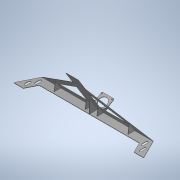
# Autodesk Inventor part: Suporte_Motor
Saved by Autodesk Inventor 2022 (Build 260153000, 153)
## iProperties
Manager: Standard
Created: 2016-02-21
Part Number: Suporte_Motor
Material: SAE 1010/1020
Document SubType Name: Modeling
Designer: Everton
Authority: Rafael Salvador
Manufacturer: Standard
Standards Organization: Custom
Density: 7.86 g/cm^3
Appearance: Steel
Mass: 19558.2 g
Surface Area: 2597.77 cm^2
Volume: 2488.33 cm^3
Author: Everton
Comments: -
Revision Number: 00
Autodesk Inventor part; units mm, degrees
ref_plane "YZ Plane" through (0, 0, 0) normal (1, 0, 0) x (0, 1, 0)
ref_plane "XZ Plane" through (0, 0, 0) normal (0, 1, 0) x (-1, 0, 0)
ref_plane "XY Plane" through (0, 0, 0) normal (0, 0, 1) x (1, 0, 0)
sketch "Sketch1" plane through (0, 0, 0) normal (0, 0, 1) x (1, 0, 0)
  line L0 (9.7407, 1114.2593) -> (159.7407, 1114.2593)
  line L1 (9.7407, 1114.2593) -> (-140.2593, 1114.2593)
  line L2 (-290.2593, 814.2593) -> (-140.2593, 1114.2593)
  line L3 (159.7407, 1114.2593) -> (459.7407, 514.2593)
  line L4 (135.0194, 1074.2593) -> (9.7407, 1074.2593)
  line L5 (9.7407, 1074.2593) -> (-115.5379, 1074.2593)
  line L6 (-115.5379, 1074.2593) -> (-245.5379, 814.2593)
  line L7 (9.7407, 1114.2593) -> (159.7407, 1114.2593)
  line L8 (9.7407, 1114.2593) -> (-140.2593, 1114.2593)
  line L9 (-440.2593, 514.2593) -> (-140.2593, 1114.2593)
  line L10 (159.7407, 1114.2593) -> (309.9483, 813.8441)
  line L11 (135.0194, 1074.2593) -> (9.7407, 1074.2593)
  line L12 (9.7407, 1074.2593) -> (-115.5379, 1074.2593)
  line L13 (-115.5379, 1074.2593) -> (-245.5379, 814.2593)
  line L14 (-245.5379, 814.2593) -> (-290.2593, 814.2593)
  line L15 (265.227, 813.8441) -> (309.9483, 813.8441)
  line L16 (265.227, 813.8441) -> (135.0194, 1074.2593)
  line L17 (415.0194, 514.2593) -> (135.0194, 1074.2593)
  line L18 (-395.5379, 514.2593) -> (-440.2593, 514.2593)
  line L19 (-245.5379, 814.2593) -> (-395.5379, 514.2593)
  line L20 (-440.2593, 514.2593) -> (-395.5379, 514.2593)
  line L21 (415.0194, 514.2593) -> (459.7407, 514.2593)
  point P0 (0, 0)
  dimension "d13" = 300
  constraints: 44 end point, 4 horizontal, 2 point on line, 1 midpoint
  measures "d13" distance from line of L6.end L1
extrude "Extrusion1" add sketch "Sketch1" along normal blind 40 contours L0 L3 L15 L16 L4 L5 L6 L14 L2 L1
extrude "Extrusion3" add sketch "Sketch1" along normal blind 40 contours L3 L21 L17 L15 | L14 L19 L18 L9
sketch "Esboço5" plane through (0, 0, 0) normal (0, 0, 1) x (1, 0, 0)
  line L0 (159.7407, 1114.2593) -> (-140.2593, 1114.2593) projected
  line L1 (400, 897.6863) -> (-384.1407, 897.6863)
  line L2 (-140.2593, 1114.2593) -> (-440.2593, 514.2593) projected
  line L3 (-248.5458, 897.6863) -> (-293.2671, 808.2435)
  line L4 (-395.5379, 514.2593) -> (-115.5379, 1074.2593) projected
  line L5 (-203.8244, 897.6863) -> (-248.5458, 808.2435)
  line L6 (-248.5458, 808.2435) -> (-293.2671, 808.2435)
  line L7 (135.0194, 1074.2593) -> (415.0194, 514.2593) projected
  line L8 (223.3059, 897.6863) -> (268.0272, 808.2435)
  line L9 (459.7407, 514.2593) -> (159.7407, 1114.2593) projected
  line L10 (268.0272, 897.6863) -> (312.7486, 808.2435)
  line L11 (312.7486, 808.2435) -> (268.0272, 808.2435)
  line L12 (-248.5458, 897.6863) -> (312.7486, 897.6863)
  line L13 (312.7486, 897.6863) -> (312.7486, 1190.7632)
  line L14 (312.7486, 1190.7632) -> (-248.5458, 1190.7632)
  line L15 (-248.5458, 1190.7632) -> (-248.5458, 897.6863)
  line L16 (-440.2593, 514.2593) -> (459.7407, 514.2593)
  line L17 (459.7407, 514.2593) -> (459.7407, 808.2435)
  line L18 (459.7407, 808.2435) -> (-440.2593, 808.2435)
  line L19 (-440.2593, 808.2435) -> (-440.2593, 514.2593)
  point P0 (0, 0)
  dimension "d26" = 100
  dimension "d27" = 100
  dimension "d28" = 100
  dimension "d29" = 100
  constraints: 30 end point, 12 point on line, 4 parallel, 3 horizontal, 2 perpendicular
  measures "d26" distance of L3.start L3.end
  measures "d27" distance of L5.start L5.end
  measures "d28" distance of L8.start L8.end
  measures "d29" distance of L10.start L10.end
extrude "Extrusão5" cut sketch "Esboço5" along normal mid plane 100 contours L9 L1 L2 L0 | L0 L2 L15 L14 L13 L1 L9 | L18 L17 L9 | L9 L16 L7 L11 | L6 L4 L16 L2 | L2 L19 L18 | L7 L16 L4 L18
sketch "Esboço6" plane through (0, 0, 0) normal (1, 0, 0) x (0, 1, 0)
  line L0 (897.6863, 40) -> (897.6863, 0) projected
  line L1 (808.2435, 0) -> (808.2435, 40) projected
  line L2 (897.6863, 0) -> (808.2435, 0)
  line L3 (808.2435, 0) -> (808.2435, 1.5)
  line L4 (808.2435, 1.5) -> (897.6863, 1.5)
  line L5 (897.6863, 1.5) -> (897.6863, 0)
  line L6 (808.2435, 1.5) -> (899.6472, 1.5)
  line L7 (899.6472, 1.5) -> (899.6472, 42.2071)
  line L8 (899.6472, 42.2071) -> (808.2435, 42.2071)
  line L9 (808.2435, 42.2071) -> (808.2435, 1.5)
  point P0 (0, 0)
  dimension "d32" = 1.5
  constraints: 16 end point, 4 parallel, 2 horizontal, 2 perpendicular, 1 point on line
  measures "d32" distance of L2.end L3.end
extrude "Extrusão6" cut sketch "Esboço6" along normal mid plane 1000 contours L4 L1 L9 L8 L7 L6
sketch "Esboço28" plane through (0, 0, 0) normal (0, 0, 1) x (1, 0, 0)
  line L0 (223.3059, 897.6863) -> (268.0272, 897.6863) projected
  line L1 (268.0272, 897.6863) -> (253.0272, 897.6863)
  line L2 (28.5, 847.4167) -> (268.0272, 897.6862) projected
  line L3 (268.0272, 897.6862) -> (258.0272, 897.6863)
  line L4 (258.0272, 897.6863) -> (258.0272, 882.6863)
  line L5 (258.0272, 882.6863) -> (258.0272, 877.6863)
  arc A0 (263.0272, 877.6863) -> (253.0272, 877.6863) centre (258.0272, 877.6863) ccw
  line L6 (258.0272, 852.6863) -> (258.0272, 857.6863)
  arc A1 (253.0272, 857.6863) -> (263.0272, 857.6863) centre (258.0272, 857.6863) ccw
  line L7 (263.0272, 877.6863) -> (263.0272, 857.6863)
  line L8 (253.0272, 877.6863) -> (253.0272, 857.6863)
  line L9 (-248.5458, 897.6862) -> (-28.5, 847.8855) projected
  line L10 (-248.5458, 897.6862) -> (-238.5458, 897.6862)
  line L11 (-203.8244, 897.6862) -> (-248.5458, 897.6862) projected
  line L12 (-238.5458, 897.6862) -> (-238.5458, 882.6862)
  line L13 (-238.5458, 882.6862) -> (-238.5458, 877.6862)
  line L14 (-238.5458, 862.6862) -> (-238.5458, 857.6862)
  line L15 (-238.5458, 857.6862) -> (-238.5458, 852.6862)
  arc A2 (-243.5458, 857.6862) -> (-233.5458, 857.6862) centre (-238.5458, 857.6862) ccw
  arc A3 (-233.5458, 877.6862) -> (-243.5458, 877.6862) centre (-238.5458, 877.6862) ccw
  line L16 (-233.5458, 877.6862) -> (-233.5458, 857.6862)
  line L17 (-243.5458, 877.6862) -> (-243.5458, 857.6862)
  line L18 (258.0272, 882.6863) -> (258.0272, 872.6863)
  line L19 (258.0272, 862.6863) -> (258.0272, 852.6863)
  line L20 (268.0272, 808.2435) -> (223.3059, 897.6863) projected
  line L21 (268.0272, 808.2435) -> (278.0272, 808.2435)
  line L22 (312.7486, 808.2435) -> (268.0272, 808.2435) projected
  line L23 (278.0272, 808.2435) -> (278.0272, 813.2435)
  line L24 (278.0272, 813.2435) -> (278.0272, 823.2435)
  line L25 (278.0272, 823.2435) -> (278.0272, 828.2435)
  line L26 (278.0272, 848.2435) -> (278.0272, 853.2435)
  arc A4 (283.0272, 848.2435) -> (273.0272, 848.2435) centre (278.0272, 848.2435) ccw
  arc A5 (273.0272, 828.2435) -> (283.0272, 828.2435) centre (278.0272, 828.2435) ccw
  line L27 (283.0272, 848.2435) -> (283.0272, 828.2435)
  line L28 (273.0272, 848.2435) -> (273.0272, 828.2435)
  line L29 (278.0272, 828.2435) -> (278.0272, 833.2435)
  line L30 (278.0272, 843.2435) -> (278.0272, 848.2435)
  line L31 (-293.2671, 808.2435) -> (-283.2671, 808.2435)
  line L32 (-248.5458, 808.2435) -> (-258.5458, 808.2435)
  line L33 (-248.5458, 808.2435) -> (268.0272, 808.2435) projected
  line L34 (-258.5458, 808.2435) -> (-258.5458, 823.2435)
  line L35 (-258.5458, 823.2435) -> (-258.5458, 828.2435)
  line L36 (-258.5458, 848.2435) -> (-258.5458, 853.2435)
  arc A6 (-253.5458, 848.2435) -> (-263.5458, 848.2435) centre (-258.5458, 848.2435) ccw
  arc A7 (-263.5458, 828.2435) -> (-253.5458, 828.2435) centre (-258.5458, 828.2435) ccw
  line L37 (-253.5458, 848.2435) -> (-253.5458, 828.2435)
  line L38 (-263.5458, 848.2435) -> (-263.5458, 828.2435)
  line L39 (-258.5458, 828.2435) -> (-258.5458, 833.2435)
  line L40 (-258.5458, 843.2435) -> (-258.5458, 848.2435)
  point P0 (0, 0)
  dimension "d126" = 10
  dimension "d127" = 15
  dimension "d128" = 30
  dimension "d129" = 5
  dimension "d130" = 10
  dimension "d131" = 5
  dimension "d132" = 10
  dimension "d133" = 10
  dimension "d134" = 15
  dimension "d135" = 5
  dimension "d136" = 20
  dimension "d137" = 5
  dimension "d138" = 10
  dimension "d139" = 10
  dimension "d140" = 10
  dimension "d143" = 5
  dimension "d144" = 20
  dimension "d145" = 5
  dimension "d146" = 10
  dimension "d147" = 10
  dimension "d149" = 10
  dimension "d151" = 15
  dimension "d152" = 20
  dimension "d153" = 5
  dimension "d154" = 10
  dimension "d155" = 10
  constraints: 68 end point, 20 point on circle, 13 point on line, 8 centre point, 8 coincident, 6 tangent, 4 vertical, 3 perpendicular, 2 midpoint, 1 parallel
  measures "d126" distance of L2.end L3.end
  measures "d127" distance of L3.end L4.end
  measures "d128" distance of L4.end L6.start
  measures "d129" distance of L4.end L5.end
  measures "d130" diameter of A0
  measures "d131" distance of L6.start L6.end
  measures "d132" diameter of A1
  measures "d133" distance of L9.start L10.end
  measures "d134" distance of L10.end L12.end
  measures "d135" distance of L12.end L13.end
  measures "d136" distance of L13.end L14.end
  measures "d137" distance of L14.end L15.end
  measures "d138" diameter of A2
  measures "d139" diameter of A3
  measures "d140" distance of L20.start L21.end
  measures "d143" distance of L24.end L25.end
  measures "d144" distance of L25.end L26.start
  measures "d145" distance of L26.start L26.end
  measures "d146" diameter of A4
  measures "d147" diameter of A5
  measures "d149" distance of L32.start L32.end
  measures "d151" distance of L32.end L34.end
  measures "d152" distance of L35.end L36.start
  measures "d153" distance of L36.start L36.end
  measures "d154" diameter of A6
  measures "d155" diameter of A7
extrude "Extrusão24" cut sketch "Esboço28" along normal mid plane 1000 contours L7 A1 L8 A0 | L17 A3 L16 A2 | L27 A5 L28 A4 | L37 A7 L38 A6
sketch "Esboço35" plane through (0, 0, 0) normal (1, 0, 0) x (0, 1, 0)
  line L0 (0, -158.5228) -> (0, 0) projected
  line L1 (0, 0) -> (0, -158.5228)
  line L2 (0, -158.5228) -> (796.9187, -158.5228) projected
  line L3 (0, -158.5228) -> (796.9187, -158.5228)
  line L4 (895.5819, 0) -> (876.9102, -30) projected
  line L5 (796.9187, -158.5228) -> (895.5819, 0)
  line L6 (895.5819, 0) -> (0, 0)
  line L7 (0, 0) -> (0, -158.5228)
  constraints: 10 end point, 2 perpendicular, 1 collinear, 1 parallel, 1 vertical
extrude "Extrusão29" cut sketch "Esboço35" along normal mid plane 1000
sketch "Esboço42" plane through (0, 0, 0) normal (0, 0, 1) x (1, 0, 0)
  line L0 (223.3059, 897.6863) -> (268.0272, 808.2435) projected
  line L1 (268.0272, 808.2435) -> (223.3059, 897.6863) projected
  line L2 (223.3059, 897.6863) -> (243.1274, 858.0433)
  line L3 (-248.5458, 808.2435) -> (-203.8244, 897.6863) projected
  line L4 (-203.8258, 897.6835) -> (-223.8244, 857.6863)
  line L5 (-203.8244, 897.6863) -> (-248.5458, 808.2435) projected
  line L6 (-203.8244, 897.6863) -> (223.3059, 897.6863)
  line L7 (223.3059, 857.6863) -> (243.3059, 857.6863)
  line L8 (243.3059, 857.6863) -> (-223.8244, 857.6863)
  line L9 (243.3059, 857.6863) -> (223.3059, 897.6863)
  point P0 (0, 0)
  point P1 (224.3581, 895.5819)
  point P2 (-204.8766, 895.5819)
  point P3 (-203.8258, 897.6835)
  dimension "d208" = 40
  constraints: 12 end point, 4 collinear, 3 point on line, 2 horizontal
  measures "d208" distance of L0.start L7.start
extrude "Extrusão33" add sketch "Esboço42" along normal blind 1.5
sketch "Esboço67" plane through (0, 0, 0) normal (0, 1, 0) x (-1, 0, 0)
  line L0 (248.5458, 0) -> (-268.0272, 0) projected
  line L1 (0, 0) -> (248.5458, 0)
  line L2 (-312.7486, 0) -> (-268.0272, 0) projected
  line L3 (248.5458, 0) -> (-268.0272, 0)
  line L4 (0, 0) -> (248.546, 0)
  line L5 (248.546, 0) -> (-9.7405, 0)
  line L6 (-9.7405, 0) -> (-9.7405, 130)
  line L7 (248.5458, 1.5) -> (248.5458, 0) projected
  line L8 (248.5458, 1.5) -> (-268.0272, 1.5) projected
  line L9 (216.6373, 1.5) -> (248.5458, 1.5)
  line L10 (-268.0272, 1.5) -> (-250.4929, 1.5)
  line L11 (-9.7407, 1.5) -> (18.7593, 1.5)
  line L12 (18.7593, 1.5) -> (-38.2407, 1.5)
  line L13 (-38.2407, 1.5) -> (-38.2407, 193.5)
  line L14 (-38.2407, 193.5) -> (18.7593, 193.5)
  line L15 (18.7593, 193.5) -> (18.7593, 1.5)
  line L16 (248.5458, 1.5) -> (203.8418, 1.5)
  line L17 (203.8418, 1.5) -> (-9.7405, 130)
  line L18 (-268.0272, 1.5) -> (-223.3232, 1.5)
  line L19 (-223.3232, 1.5) -> (-9.7405, 130)
  line L20 (248.5458, 1.5) -> (-9.7405, 156.3842)
  line L21 (-268.0272, 1.5) -> (-312.7486, 1.5) projected
  line L22 (-9.7405, 156.3842) -> (-268.0272, 1.5)
  line L23 (146.5111, 1.5) -> (146.5111, 31.5)
  line L24 (146.5111, 31.5) -> (153.9782, 31.5)
  line L25 (-173.4596, 31.5) -> (146.5111, 31.5)
  line L26 (153.9782, 31.5) -> (203.8418, 1.5)
  line L27 (203.8418, 1.5) -> (-223.3232, 1.5)
  line L28 (-223.3232, 1.5) -> (-173.4596, 31.5)
  point P0 (-38.2407, 139.2938)
  point P1 (-38.2407, 112.8531)
  point P2 (18.7593, 139.294)
  point P3 (18.7593, 112.8534)
  point P4 (18.7593, 31.5)
  point P5 (-38.2407, 31.5)
  dimension "d288" = 516.573
  dimension "d290" = 258.2865
  dimension "d291" = 130
  dimension "d292" = 28.5
  dimension "d293" = 57
  dimension "d294" = 192
  dimension "d297" = 44.704
  dimension "d298" = 44.704
  dimension "d305" = 30
  constraints: 48 end point, 9 point on line, 6 collinear, 3 parallel, 3 perpendicular, 1 horizontal, 1 midpoint, 1 vertical
  measures "d288" distance of L0.start L0.end
  measures "d290" distance of L4.end L5.end
  measures "d291" distance of L5.end L6.end
  measures "d292" distance of L11.start L11.end
  measures "d293" distance of L13.end L14.end
  measures "d294" distance of L12.end L13.end
  measures "d297" distance of L7.start L16.end
  measures "d298" distance of L8.end L18.end
  measures "d305" distance of L23.start L23.end
extrude "Extrusão54" add sketch "Esboço67" along normal blind 1000 contours L8 L17 L15 L20 | L20 L22 L13 L14 L15 | L15 L17 L19 L13 L22 L20 | L8 L13 L25 L6 | L6 L25 L15 L8 | L8 L23 L24 L17 | L15 L25 L6 L17 | L25 L13 L19 L6 | L15 L25 L23 L8 | L8 L19 L25 L13 | L13 L19 L8 L22
sketch "Esboço69" plane through (0, 0, 0) normal (1, 0, 0) x (0, 1, 0)
  line L0 (897.6863, 1.5) -> (1000, 1.5) projected
  line L1 (1000, 1.5) -> (897.6863, 1.5)
  line L2 (1000, 112.8531) -> (1000, 1.5) projected
  line L3 (1000, 1.5) -> (1000, 193.5)
  line L4 (1000, 193.5) -> (897.6863, 193.5)
  line L5 (0, 193.5) -> (1000, 193.5) projected
  line L6 (897.6863, 0) -> (897.6863, 193.5)
  line L7 (897.6863, 0) -> (897.6863, 193.5)
  line L8 (897.6863, 1.5) -> (897.6863, 0) projected
  line L9 (897.6863, 1.5) -> (897.6863, 193.5)
  line L10 (897.6863, 193.5) -> (777.6888, 193.5)
  line L11 (777.6888, 193.5) -> (897.6863, 1.5)
  line L12 (895.4877, 5.0178) -> (894.2157, 4.2228)
  line L13 (789.1746, 175.1222) -> (787.9026, 174.3273)
  line L14 (808.2435, 1.5) -> (897.6863, 1.5) projected
  line L15 (0, 1.5) -> (857.6863, 1.5) projected
  line L16 (894.8517, 1.5) -> (0, 1.5)
  line L17 (0, 139.294) -> (0, 193.5) projected
  line L18 (0, 1.5) -> (0, 193.5)
  line L19 (0, 193.5) -> (777.6888, 193.5)
  line L20 (775.9199, 193.5) -> (895.9174, 1.5)
  point P0 (0, 0)
  point P1 (895.9174, 1.5)
  dimension "d300" = 119.9975
  dimension "d301" = 1.5
  dimension "d302" = 1.5
  constraints: 28 end point, 7 point on line, 6 perpendicular, 2 collinear, 1 horizontal, 1 parallel
  measures "d300" distance of L4.end L10.end
  measures "d301" distance of L12.start L12.end
  measures "d302" distance of L13.start L13.end
extrude "Extrusão55" cut sketch "Esboço69" along normal mid plane 1000 contours L6 L4 L3 L2 L0 | L11 L5 L6 | L14 L15 L18 L17 L5 L20
sketch "Esboço70" plane through (0, 0, 0) normal (0, 1, 0) x (-1, 0, 0)
  line L0 (-38.2407, 112.8531) -> (-38.2407, 31.5) projected
  line L1 (18.7593, 0) -> (-38.2407, 0)
  line L2 (-38.2407, 0) -> (-38.2407, 57)
  line L3 (-38.2407, 57) -> (18.7593, 57)
  line L4 (18.7593, 57) -> (18.7593, 0)
  point P0 (0, 0)
  point P1 (-38.2407, 31.5)
  dimension "d306" = 57
  constraints: 8 end point, 2 parallel, 1 horizontal, 1 perpendicular, 1 point on line
  measures "d306" distance of L1.end L2.end
extrude "Extrusão56" add sketch "Esboço70" along normal blind 1000
sketch "Esboço71" plane through (0, 0, 0) normal (1, 0, 0) x (0, 1, 0)
  line L0 (811.5668, 139.294) -> (897.6863, 1.5) projected
  line L1 (897.6863, 1.5) -> (946.0224, 31.7095)
  line L2 (946.0224, 31.7095) -> (944.9625, 33.4055)
  line L3 (944.9625, 33.4055) -> (896.6263, 3.196)
  line L4 (897.6863, 1.5) -> (862.9995, 57)
  line L5 (878.9367, 31.5) -> (828.0919, 112.8534) projected
  line L6 (862.9995, 57) -> (1000, 57) projected
  line L7 (862.9995, 57) -> (1000, 57)
  line L8 (1000, 57) -> (1000, 0) projected
  line L9 (1000, 57) -> (1000, 0)
  line L10 (1000, 0) -> (897.6863, 0)
  line L11 (897.6863, 1.5) -> (895.9174, 1.5) projected
  line L12 (897.6863, 0) -> (897.6863, 1.5)
  line L13 (897.6863, 1.5) -> (896.6263, 3.196)
  line L14 (0, 0) -> (857.6863, 0) projected
  line L15 (0, 0) -> (0, 57)
  line L16 (0, 57) -> (861.2306, 57)
  line L17 (826.323, 112.8534) -> (877.1678, 31.5) projected
  line L18 (0, 57) -> (861.2306, 57) projected
  line L19 (895.9174, 1.5) -> (877.1678, 31.5) projected
  line L20 (861.2306, 57) -> (895.9174, 1.5)
  line L21 (895.9174, 1.5) -> (808.2429, 1.5)
  line L22 (808.2429, 1.5) -> (808.2429, 0)
  line L23 (857.6863, 0) -> (808.2435, 0) projected
  line L24 (0, 0) -> (808.2435, 0)
  dimension "d310" = 57
  dimension "d311" = 2
  constraints: 30 end point, 6 perpendicular, 6 point on line, 3 horizontal, 2 collinear, 1 vertical
  measures "d310" distance of L0.end L1.end
  measures "d311" distance of L1.end L2.end
extrude "Extrusão57" cut sketch "Esboço71" along normal mid plane 1000 contours L6 L8 L10 L12 L1 L2 L3 L0 | L15 L16 L17 L19 L21 L22 L14
sketch "Esboço72" plane through (0, 0, 0) normal (0, 0, 1) x (1, 0, 0)
  line L0 (38.2407, 857.6863) -> (38.2407, 808.2429) projected
  line L1 (38.2407, 857.6863) -> (-20.8185, 857.6863)
  line L2 (-20.8185, 857.6863) -> (-20.8185, 805.8678)
  line L3 (-20.8185, 805.8678) -> (38.2407, 805.8678)
  line L4 (38.2407, 805.8678) -> (38.2407, 857.6863)
  point P0 (0, 0)
  constraints: 8 end point, 2 parallel, 1 horizontal, 1 perpendicular
extrude "Extrusão58" cut sketch "Esboço72" along normal blind 5
sketch "Esboço73" plane through (0, 0, 0) normal (1, 0, 0) x (0, 1, 0)
  line L0 (811.5668, 139.294) -> (897.6863, 1.5) projected
  line L1 (896.6266, 3.1955) -> (913.5863, 13.7958)
  line L2 (896.6263, 3.196) -> (886.0265, 20.1561)
  line L3 (886.0265, 20.1561) -> (913.5863, 13.7958)
  line L4 (896.6263, 3.196) -> (897.6863, 1.5)
  line L5 (946.0224, 31.7095) -> (897.6863, 1.5) projected
  line L6 (913.5863, 13.7958) -> (916.3423, 13.1598)
  line L7 (916.3423, 13.1598) -> (897.6863, 1.5)
  line L8 (895.9174, 1.5) -> (897.6863, 1.5) projected
  line L9 (897.6863, 1.5) -> (896.6263, 3.196)
  point P0 (0, 0)
  dimension "d317" = 20
  dimension "d318" = 20
  constraints: 14 end point, 3 point on line, 2 collinear, 1 perpendicular
  measures "d317" distance of L1.start L1.end
  measures "d318" distance of L2.start L2.end
extrude "Extrusão59" add sketch "Esboço73" along normal blind 40.241
sketch "Esboço75" plane through (0, 0, 0) normal (1, 0, 0) x (0, 1, 0)
  line L0 (886.0265, 20.1561) -> (896.6263, 3.196) projected
  line L1 (886.0265, 20.1561) -> (897.6863, 1.5)
  line L2 (897.6863, 1.5) -> (886.0265, 20.1561)
  line L3 (897.6863, 1.5) -> (811.567, 139.2938) projected
  line L4 (886.0265, 20.1561) -> (916.3423, 13.1598)
  line L5 (913.5863, 13.7958) -> (886.0265, 20.1561) projected
  line L6 (897.6863, 1.5) -> (946.0224, 31.7095) projected
  line L7 (916.3423, 13.1598) -> (897.6863, 1.5)
  point P0 (0, 0)
  point P1 (896.6263, 3.196)
  constraints: 8 end point, 3 collinear, 1 perpendicular
extrude "Extrusão60" add sketch "Esboço75" against normal blind 20.759
sketch "Esboço79" plane through (0, 0, 0) normal (1, 0, 0) x (0, 1, 0)
  line L0 (897.6863, 1.5) -> (896.6263, 3.196)
  line L1 (896.6263, 3.196) -> (913.5863, 13.7958)
  line L2 (897.6863, 1.5) -> (916.3423, 13.1598) projected
  line L3 (886.027, 20.1552) -> (896.6263, 3.196)
  line L4 (896.6263, 3.196) -> (885.2658, 21.3731)
  line L5 (897.6863, 1.5) -> (811.567, 139.2938) projected
  line L6 (885.2658, 21.3731) -> (914.5125, 14.3747)
  line L7 (914.5125, 14.3747) -> (896.6263, 3.196)
  point P0 (0, 0)
  dimension "d327" = 2
  constraints: 12 end point, 2 parallel, 2 point on line, 1 collinear
  measures "d327" distance of L0.start L0.end
extrude "Extrusão63" cut sketch "Esboço79" against normal blind 18.759
sketch "Esboço80" plane through (0, 0, 0) normal (1, 0, 0) x (0, 1, 0)
  line L0 (897.6863, 1.5) -> (896.6263, 3.196)
  line L1 (897.6863, 1.5) -> (811.567, 139.2938) projected
  line L2 (896.6263, 3.196) -> (914.6531, 14.4625)
  line L3 (914.6531, 14.4625) -> (885.0966, 21.6439)
  line L4 (885.0966, 21.6439) -> (896.6263, 3.196)
  point P0 (0, 0)
  dimension "d330" = 2
  constraints: 8 end point, 2 point on line, 1 collinear, 1 perpendicular
  measures "d330" distance of L0.start L0.end
extrude "Extrusão64" cut sketch "Esboço80" along normal blind 38.241
sketch "Esboço82" plane through (0, 0, 0) normal (1, 0, 0) x (0, 1, 0)
  line L0 (895.9174, 1.5) -> (897.6863, 1.5) projected
  line L1 (895.9174, 1.5) -> (872.0678, 39.6601)
  line L2 (895.9174, 1.5) -> (809.7979, 139.294) projected
  line L3 (895.9174, 1.5) -> (865.9174, 1.5)
  line L4 (808.2435, 1.5) -> (897.6863, 1.5) projected
  line L5 (865.9174, 1.5) -> (872.0678, 39.6601)
  point P0 (0, 0)
  dimension "d336" = 45
  dimension "d337" = 30
  constraints: 6 end point, 2 point on line
  measures "d336" distance of L0.start L1.end
  measures "d337" distance of L0.start L3.end
extrude "Extrusão66" add sketch "Esboço82" along normal blind 183
sketch "Esboço84" plane through (0, 0, 0) normal (1, 0, 0) x (0, 1, 0)
  line L0 (872.0678, 39.6601) -> (895.9174, 1.5) projected
  line L1 (895.9174, 1.5) -> (865.9174, 1.5)
  line L2 (865.9174, 1.5) -> (872.0678, 39.6601)
  line L3 (809.7981, 139.2938) -> (895.9174, 1.5) projected
  line L4 (872.0678, 39.6601) -> (895.9174, 1.5)
  point P0 (0, 0)
  constraints: 6 end point, 1 point on line
extrude "Extrusão67" cut sketch "Esboço84" along normal blind 181
sketch "Esboço85" plane through (0, 0, 0) normal (1, 0, 0) x (0, 1, 0)
  line L0 (895.9174, 1.5) -> (872.0678, 39.6602)
  line L1 (826.323, 112.8534) -> (877.1678, 31.5) projected
  line L2 (865.9174, 1.5) -> (895.9174, 1.5) projected
  line L3 (872.0678, 39.6602) -> (865.9174, 1.5)
  line L4 (865.9174, 1.5) -> (895.9174, 1.5)
  point P0 (0, 0)
  constraints: 6 end point, 1 collinear, 1 point on line
extrude "Extrusão68" add sketch "Esboço85" against normal blind 163.518
sketch "Esboço86" plane through (0, 0, 0) normal (1, 0, 0) x (0, 1, 0)
  line L0 (872.0678, 39.6602) -> (865.9174, 1.5) projected
  line L1 (872.0678, 39.6602) -> (826.323, 112.8534) projected
  line L2 (865.9174, 1.5) -> (872.0678, 39.6602)
  line L3 (872.0678, 39.6602) -> (895.9174, 1.5)
  line L4 (895.9174, 1.5) -> (865.9174, 1.5) projected
  line L5 (865.9174, 1.5) -> (895.9174, 1.5)
  point P0 (0, 0)
  constraints: 6 end point, 2 collinear
extrude "Extrusão69" cut sketch "Esboço86" against normal blind 161.518
sketch "Esboço87" plane through (0, 0, 0) normal (1, 0, 0) x (0, 1, 0)
  line L0 (865.9174, 1.5) -> (895.9174, 1.5) projected
  line L1 (895.9174, 1.5) -> (872.0678, 39.6602) projected
  line L2 (895.9174, 1.5) -> (872.0678, 39.6602)
  line L3 (872.0678, 39.6602) -> (865.9174, 1.5)
  line L4 (865.9174, 1.5) -> (895.9174, 1.5)
  point P0 (0, 0)
  constraints: 6 end point, 1 collinear, 1 horizontal
extrude "Extrusão70" add sketch "Esboço87" along normal blind 38.241
sketch "Esboço88" plane through (0, 0, 0) normal (1, 0, 0) x (0, 1, 0)
  line L0 (895.9174, 1.5) -> (872.0678, 39.6602)
  line L1 (895.9174, 1.5) -> (865.9174, 1.5)
  line L2 (865.9174, 1.5) -> (872.0678, 39.6602)
  line L3 (872.0678, 39.6602) -> (895.9174, 1.5) projected
  line L4 (872.0678, 39.6602) -> (895.9174, 1.5)
  line L5 (895.9174, 1.5) -> (865.9174, 1.5)
  line L6 (865.9174, 1.5) -> (895.9174, 1.5) projected
  point P0 (0, 0)
  constraints: 10 end point, 2 collinear, 1 horizontal
extrude "Extrusão71" cut sketch "Esboço88" along normal blind 36.241
sketch "Esboço89" plane through (0, 0, 0) normal (1, 0, 0) x (0, 1, 0)
  line L0 (865.9174, 1.5) -> (895.9174, 1.5) projected
  line L1 (895.9174, 1.5) -> (872.0678, 39.6595)
  line L2 (872.0678, 39.6595) -> (865.9176, 1.5)
  line L3 (865.9176, 1.5) -> (895.9174, 1.5)
  point P0 (0, 0)
  constraints: 6 end point, 1 horizontal
extrude "Extrusão72" add sketch "Esboço89" against normal blind 18.759
sketch "Esboço90" plane through (0, 0, 0) normal (1, 0, 0) x (0, 1, 0)
  line L0 (872.0678, 39.6595) -> (895.9174, 1.5) projected
  line L1 (895.9174, 1.5) -> (872.0678, 39.6595)
  line L2 (865.9174, 1.5) -> (895.9174, 1.5) projected
  line L3 (872.0678, 39.6595) -> (865.9174, 1.5)
  line L4 (865.9174, 1.5) -> (895.9174, 1.5)
  point P0 (0, 0)
  constraints: 6 end point, 1 collinear, 1 horizontal
extrude "Extrusão73" cut sketch "Esboço90" against normal blind 16.759
sketch "Esboço91" plane through (0, 0, 0) normal (1, 0, 0) x (0, 1, 0)
  line L0 (872.0678, 39.6601) -> (895.9174, 1.5) projected
  line L1 (895.9174, 1.5) -> (855.9174, 1.5)
  line L2 (877.6863, 1.5) -> (857.6863, 1.5) projected
  line L3 (855.9174, 1.5) -> (855.9174, 65.5013)
  line L4 (877.1678, 31.5) -> (826.323, 112.8534) projected
  line L5 (855.9174, 65.5013) -> (895.9174, 1.5)
  point P0 (0, 0)
  dimension "d355" = 40
  constraints: 6 end point, 2 collinear, 1 point on line, 1 vertical
  measures "d355" distance of L0.end L1.end
extrude "Extrusão74" add sketch "Esboço91" along normal blind 10.741
sketch "Esboço93" plane through (0, 0, 0) normal (1, 0, 0) x (0, 1, 0)
  line L0 (895.9174, 1.5) -> (872.0678, 39.6602) projected
  line L1 (895.9174, 1.5) -> (853.3346, 69.634)
  line L2 (853.3346, 69.634) -> (853.3346, 1.5)
  line L3 (897.6863, 1.5) -> (808.2435, 1.5) projected
  line L4 (853.3346, 1.5) -> (895.9174, 1.5)
  line L5 (808.2435, 0) -> (897.6863, 0) projected
  point P0 (0, 0)
  constraints: 6 end point, 1 collinear, 1 parallel, 1 point on line, 1 vertical
extrude "Extrusão76" cut sketch "Esboço93" along normal blind 8.741
sketch "Esboço94" plane through (0, 0, 0) normal (1, 0, 0) x (0, 1, 0)
  line L0 (897.6863, 1.5) -> (808.2435, 1.5) projected
  line L1 (855.9167, 1.5) -> (858.2357, 1.5)
  line L2 (858.2357, 1.5) -> (858.24, 61.7852)
  line L3 (877.1678, 31.5) -> (826.3232, 112.8531) projected
  line L4 (858.24, 61.7852) -> (855.9174, 65.5013)
  line L5 (855.9174, 65.5013) -> (855.9174, 1.5) projected
  line L6 (855.9174, 65.5013) -> (855.9174, 1.5)
  point P0 (0, 0)
  dimension "d362" = 2.319
  constraints: 8 end point, 4 point on line, 1 vertical
  measures "d362" distance of L1.start L1.end
extrude "Extrusão77" cut sketch "Esboço94" along normal mid plane 8741
sketch "Esboço95" plane through (-18.7593, 944.9625, 33.4055) normal (0, -0.529991, 0.8480033) x (1, 0, 0)
  line L0 (0, 0) -> (57, 0) projected
  line L1 (0, -37) -> (0, 0) projected
  point P0 (18.7593, -819.0359)
  point P1 (28.5, -28.5)
  dimension "d372" = 28.5
  dimension "d373" = 28.5
  measures "d372" distance from line of L0 point (28.5, -28.5)
  measures "d373" distance from line of L1 point (28.5, -28.5)
hole "Furo7" at (9.7407, 920.7944, 18.3007) direction (0, 0.529991, -0.8480033) diameter 40 depth 14.2 start extended yes
sketch "Esboço96" plane through (-18.7593, 944.9625, 33.4055) normal (0, -0.529991, 0.8480033) x (1, 0, 0)
  line L0 (0, 0) -> (57, 0) projected
  line L1 (0, -37) -> (0, 0) projected
  line L2 (57, 0) -> (57, -37) projected
  line L3 (57.0003, -37) -> (57.0003, -57) projected
  line L4 (57, -57) -> (0, -57) projected
  line L5 (0.0003, -57) -> (0.0003, -37) projected
  point P0 (18.7593, -819.0359)
  point P1 (5.0003, -52)
  point P2 (52.0003, -52)
  point P3 (52, -5)
  point P4 (5, -5)
  dimension "d381" = 5
  dimension "d382" = 5
  dimension "d383" = 5
  dimension "d384" = 5
  dimension "d385" = 5
  dimension "d386" = 5
  dimension "d387" = 5
  dimension "d388" = 5
  measures "d381" distance from line of L0 point (5, -5)
  measures "d382" distance from line of L1 point (5, -5)
  measures "d383" distance from line of L2 point (52, -5)
  measures "d384" distance from line of L0 point (52, -5)
  measures "d385" distance from line of L3 point (52, -52)
  measures "d386" distance from line of L4 point (52, -52)
  measures "d387" distance from line of L5 point (5, -52)
  measures "d388" distance from line of L4 point (5, -52)
hole "Furo8" at (-13.759, 900.8663, 5.846) at (33.241, 900.8663, 5.846) at (33.2407, 940.7224, 30.7555) at (-13.7593, 940.7224, 30.7555) direction (0, 0.529991, -0.8480033) diameter 4.4587 depth 12.8 start extended yes thread size "M5x0.5" class "6H" standard "ANSI Metric M Profile"
chamfer "Chanfro1" distance 2 angle 45 2 edges at (-18.7593, 945.4925, 32.5575) (38.2407, 945.4925, 32.5575)
fillet "Arredondamento4" radius 2 8 edges at (-18.7593, 776.8043, 193.5) (38.2407, 776.8043, 193.5) (312.7486, 808.2435, 0.75) (268.0272, 808.2435, 0.75) (268.0272, 897.6863, 0.75) (-248.5458, 897.6863, 0.75) (-293.2671, 808.2435, 0.75) (-248.5458, 808.2435, 0.75)
body "Solid1"
